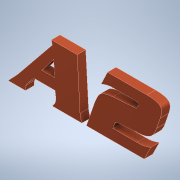
# Autodesk Inventor part: A2
Saved by Autodesk Inventor 2021 (Build 250183000, 183)
## iProperties
Created: 2021-03-21
Part Number: A2
Material: Copper, Wrought
Document SubType Name: Modeling
Designer: TieuBinh
Density: 8.94 g/cm^3
Appearance: Copper - Satin
Author: TieuBinh
Autodesk Inventor part; units mm, degrees
ref_plane "YZ Plane" through (0, 0, 0) normal (1, 0, 0) x (0, 1, 0)
ref_plane "XZ Plane" through (0, 0, 0) normal (0, 1, 0) x (-1, 0, 0)
ref_plane "XY Plane" through (0, 0, 0) normal (0, 0, 1) x (1, 0, 0)
sketch "Sketch 1" plane through (0, 0, 0) normal (0, 0, 1) x (1, 0, 0)
  line L0 (-474.0154, 284.8231) -> (44.1949, 284.8231) construction
  line L1 (44.1949, 284.8231) -> (44.1949, 84.8231) construction
  line L2 (44.1949, 84.8231) -> (-474.0154, 84.8231) construction
  line L3 (-474.0154, 84.8231) -> (-474.0154, 284.8231) construction
  line L4 (-235.3969, 284.8231) -> (-225.5068, 111.1967)
  spline S0 degree 2 poles (-225.5068, 111.1967) (-224.5649, 100.3647) (-219.2274, 84.8231) knots 0 0 0 1 1 1
  line L5 (-219.2274, 84.8231) -> (-322.995, 84.8231)
  spline S1 degree 2 poles (-322.995, 84.8231) (-314.6748, 94.5562) (-312.477, 100.9926) knots 0 0 0 1 1 1
  spline S2 degree 2 poles (-312.477, 100.9926) (-309.6512, 109.4699) (-312.477, 131.7619) (-313.1049, 137.2564) knots 0 0 0 1 2 2 2
  line L6 (-313.1049, 137.2564) -> (-388.4581, 137.2564)
  line L7 (-388.4581, 137.2564) -> (-408.2384, 112.6096)
  spline S3 degree 2 poles (-408.2384, 112.6096) (-410.7501, 109.3129) (-414.6748, 103.9754) (-415.4597, 101.1496) knots 0 0 0 1 2 2 2
  spline S4 degree 2 poles (-415.4597, 101.1496) (-416.4016, 98.6378) (-416.7156, 92.3584) (-417.3435, 84.8231) knots 0 0 0 1 2 2 2
  line L8 (-417.3435, 84.8231) -> (-477.7831, 84.8231)
  spline S5 degree 2 poles (-477.7831, 84.8231) (-466.6371, 97.068) (-448.7407, 115.2783) (-440.4205, 125.3254) knots 0 0 0 1 2 2 2
  line L9 (-440.4205, 125.3254) -> (-322.995, 270.2234)
  spline S6 degree 2 poles (-322.995, 270.2234) (-323.937, 275.5609) (-325.9778, 284.8231) knots 0 0 0 1 1 1
  line L10 (-325.9778, 284.8231) -> (-235.3969, 284.8231)
  line L11 (-317.9715, 228.9361) -> (-360.5147, 174.462)
  line L12 (-360.5147, 174.462) -> (-314.6748, 174.462)
  line L13 (-314.6748, 174.462) -> (-317.9715, 228.9361)
  spline S7 degree 2 poles (9.501, 284.8231) (41.0552, 284.8231) (66.9579, 267.8686) (56.5968, 237.7273) knots 0 0 0 1 2 2 2
  line L14 (56.5968, 237.7273) -> (43.8809, 200.2077)
  spline S8 degree 2 poles (43.8809, 200.2077) (34.4618, 172.2642) (1.9657, 153.7399) (-26.2917, 153.7399) knots 0 0 0 1 2 2 2
  line L15 (-26.2917, 153.7399) -> (-87.6732, 149.3443)
  spline S9 degree 2 poles (-87.6732, 149.3443) (-98.8192, 148.2454) (-102.1159, 146.3615) (-103.9997, 141.338) knots 0 0 0 1 2 2 2
  line L16 (-103.9997, 141.338) -> (-110.2792, 122.6567)
  line L17 (-110.2792, 122.6567) -> (-25.9778, 122.6567)
  spline S10 degree 2 poles (-25.9778, 122.6567) (-11.6921, 122.6567) (5.5764, 125.6394) (23.3158, 131.7619) knots 0 0 0 1 2 2 2
  line L18 (23.3158, 131.7619) -> (0.0819, 84.8231)
  line L19 (0.0819, 84.8231) -> (-203.0578, 84.8231)
  line L20 (-203.0578, 84.8231) -> (-177.7831, 159.0774)
  spline S11 degree 2 poles (-177.7831, 159.0774) (-165.6952, 194.5562) (-143.8742, 216.0633) (-110.4362, 218.732) knots 0 0 0 1 2 2 2
  line L21 (-110.4362, 218.732) -> (-41.2054, 223.7556)
  line L22 (-41.2054, 223.7556) -> (-35.5539, 223.7556)
  spline S12 degree 2 poles (-35.5539, 223.7556) (-29.2745, 223.7556) (-24.4079, 228.1512) (-22.0531, 235.5295) knots 0 0 0 1 2 2 2
  spline S13 degree 2 poles (-22.0531, 235.5295) (-19.6983, 242.1229) (-22.5241, 246.9895) (-29.1175, 246.9895) knots 0 0 0 1 2 2 2
  line L23 (-29.1175, 246.9895) -> (-109.9652, 246.9895)
  spline S14 degree 2 poles (-109.9652, 246.9895) (-120.1693, 246.9895) (-136.3388, 243.3788) (-150.9385, 238.0413) knots 0 0 0 1 2 2 2
  line L24 (-150.9385, 238.0413) -> (-128.8035, 284.8231)
  line L25 (-128.8035, 284.8231) -> (9.501, 284.8231)
  point P0 (0, 0)
  constraints: 2 other
extrude "Extrusion1" add sketch "Sketch 1" along normal blind 30
body "Solid1"
